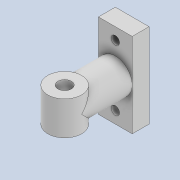
# Autodesk Inventor part: 10-06-008
Saved by Autodesk Inventor 2020 (Build 240168000, 168)
## iProperties
Created: 2019-11-09
Part Number: 10-06-008
Material: Generic
Document SubType Name: Modeling
Designer: iuliu
Density: 1 g/cm^3
Appearance: Default
Description: Suport display
Mass: 21.0778 g
Surface Area: 67.6261 cm^2
Volume: 21.0778 cm^3
Author: iuliu
Subject: 045
Autodesk Inventor part; units mm, degrees
ref_plane "YZ Plane" through (0, 0, 0) normal (1, 0, 0) x (0, 1, 0)
sketch "Sketch1" plane through (0, 0, 0) normal (0, 0, 1) x (1, 0, 0)
  line L0 (-10, 25) -> (10, 25)
  line L1 (10, 25) -> (10, -25)
  line L2 (10, -25) -> (-10, -25)
  line L3 (-10, -25) -> (-10, 25)
  circle A0 centre (0, 18) radius 2.5
  circle A1 centre (0, -18) radius 2.5
  point P0 (0, 0)
  point P1 (-10, 0)
  point P2 (0, 25)
  dimension "d0" = 20
  dimension "d1" = 50
  dimension "d2" = 5
  dimension "d3" = 7
  dimension "d4" = 7
  constraints: 8 end point, 3 vertical alignment, 2 centre point, 2 midpoint, 2 parallel, 1 equal radius, 1 horizontal, 1 horizontal alignment, 1 perpendicular
  measures "d0" distance of L0.start L0.end
  measures "d1" distance of L2.end L0.start
  measures "d2" diameter of A0
  measures "d3" distance from line of A0.centre L0
  measures "d4" distance from line of L2 A1.centre
extrude "Extrusion1" add sketch "Sketch1" along normal blind 10
ref_plane "Work Plane1" through (0, -10, 0) normal (0, 1, 0) x (-1, 0, 0)
ref_plane "Work Plane2" through (10, -25, 10) normal (-0.7071, 0, 0.7071) x (0, 1, 0)
sketch "Sketch7" plane through (10, -25, 10) normal (0, 0, 1) x (0, 1, 0)
  line L0 (50, 0) -> (0, 0) projected
  circle A0 centre (25, 10) radius 10
  line L1 (50, 20) -> (0, 20) projected
  circle A1 centre (43, 10) radius 2.5 projected
  circle A2 centre (7, 10) radius 2.5 projected
  line L2 (0, 20) -> (50, 20) projected
  line L3 (50, 20) -> (50, 0) projected
  line L4 (0, 0) -> (0, 20) projected
  point P0 (25, 10)
  point P1 (25, 20)
  dimension "d28" = 20
  dimension "d29" = 10
  constraints: 1 centre point, 1 vertical alignment, 2 other
  measures "d28" diameter of A0
  measures "d29" distance from line of L0 A0.centre
extrude "Extrusion6" add sketch "Sketch7" along normal blind 30 contours A0
sketch "Sketch8" plane through (0, 0, 0) normal (0, 1, 0) x (-1, 0, 0)
  circle A0 centre (0, 40) radius 10
  line L0 (-10, 10) -> (-10, 40) projected
  line L1 (-10, 40) -> (10, 40) projected
  line L2 (10, 40) -> (10, 10) projected
  line L3 (10, 10) -> (10, 0) projected
  line L4 (10, 0) -> (-10, 0) projected
  line L5 (-10, 0) -> (-10, 10) projected
  point P0 (0, 0)
  point P1 (25.3553, 31.2132)
  point P2 (-10, 3.7868)
  dimension "d47" = 20
  constraints: 2 coincident, 1 centre point, 1 midpoint
  measures "d47" diameter of A0
extrude "Extrusion7" add sketch "Sketch8" along normal mid plane 20 contours L1 A0 | A0 L1
sketch "Sketch9" plane through (0, 10, 40) normal (0, 1, 0) x (1, 0, 0)
  circle A0 centre (0, 0) radius 4
  circle A1 centre (0, 0) radius 10 projected
  point P0 (0, 40)
  point P1 (-3.2583, 9.4543)
  point P2 (3.2583, 9.4543)
  point P3 (-2.6421, 9.6447)
  point P4 (2.6421, 9.6447)
  point P5 (0, 10)
  point P6 (0, 10)
  dimension "d35" = 8
  constraints: 1 centre point, 1 concentric
  measures "d35" diameter of A0
extrude "Extrusion8" cut sketch "Sketch9" against normal through all contours A0
equation "\"d4\" = d3"
body "Solid1"
